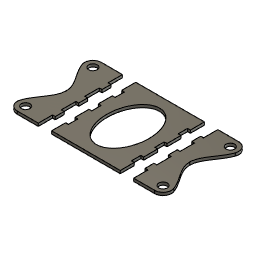
Spuhlenhalter (Autodesk Fusion 360 design; units mm, degrees)
Autodesk Fusion 360 part; units mm, degrees
sketch "Skizze1" plane through (0, 0, 0) normal (0, 1, 0) x (1, 0, 0)
  line L0 (-45, 60) -> (45, 60)
  line L1 (45, 60) -> (45, -60)
  line L2 (45, -60) -> (-45, -60)
  line L3 (-45, -60) -> (-45, 60)
  line L4 (-45, 60) -> (45, -60) construction
  line L5 (45, 60) -> (-45, -60) construction
  line L6 (-45, 60) -> (-49, 60)
  line L7 (-49, 60) -> (-49, 40)
  line L8 (-49, 40) -> (-45, 40)
  line L9 (-45, 40) -> (-45, 60)
  line L10 (-49, 26.6667) -> (-49, 6.6667)
  line L11 (-45, 6.6667) -> (-45, 26.6667)
  line L12 (-45, 26.6667) -> (-49, 26.6667)
  line L13 (-49, 6.6667) -> (-45, 6.6667)
  line L14 (-49, -6.6667) -> (-49, -26.6667)
  line L15 (-45, -26.6667) -> (-45, -6.6667)
  line L16 (-45, -6.6667) -> (-49, -6.6667)
  line L17 (-49, -26.6667) -> (-45, -26.6667)
  line L18 (-49, -40) -> (-49, -60)
  line L19 (-45, -60) -> (-45, -40)
  line L20 (-45, -40) -> (-49, -40)
  line L21 (-49, -60) -> (-45, -60)
  line L22 (0, -1.75) -> (0, -22.5)
  line L23 (45, -40) -> (49, -40)
  line L24 (45, 60) -> (49, 60)
  line L25 (45, 6.6667) -> (45, 26.6667)
  line L26 (49, -26.6667) -> (45, -26.6667)
  line L27 (49, 40) -> (45, 40)
  line L28 (49, -60) -> (45, -60)
  line L29 (45, -60) -> (45, -40)
  line L30 (45, -60) -> (45, 60)
  line L31 (45, 26.6667) -> (49, 26.6667)
  line L32 (49, 6.6667) -> (45, 6.6667)
  line L33 (49, -6.6667) -> (49, -26.6667)
  line L34 (49, 60) -> (49, 40)
  line L35 (45, -6.6667) -> (49, -6.6667)
  line L36 (49, -40) -> (49, -60)
  line L37 (45, -26.6667) -> (45, -6.6667)
  line L38 (45, 40) -> (45, 60)
  line L39 (49, 26.6667) -> (49, 6.6667)
  ellipse E0 centre (0, 0) end of major axis (0, -45) minor radius 30
  line L40 (0, 45) -> (0, -45)
  line L41 (-30, 0) -> (30, 0)
  dimension "d1" = 90
  dimension "d2" = 120
  dimension "d3" = 4
  dimension "d4" = 20
  dimension "d7" = 0
  dimension "d8" = -100
  dimension "d9" = 60
  dimension "d10" = 45
  constraint horizontal L0
  constraint perpendicular L0 L1
  constraint parallel L0 L2
  constraint parallel L1 L3
  constraint coincident L4 E0.centre
  constraint coincident L5 E0.centre
  constraint coincident E0.centre origin
  constraint horizontal L6
  constraint vertical L7
  constraint horizontal L8
  constraint vertical L9
  constraint symmetric L0.start L22 L0.end
  constraint symmetric L2.end L22 L1.end
  constraint symmetric L6.end L22 L24.end
  constraint symmetric L7.end L22 L27.start
  constraint symmetric L8.end L22 L27.end
  constraint symmetric L11.start L22 L25.start
  constraint symmetric L10.start L22 L31.end
  constraint symmetric L10.end L22 L32.start
  constraint symmetric L11.end L22 L25.end
  constraint symmetric L15.start L22 L26.end
  constraint symmetric L14.start L22 L33.start
  constraint symmetric L14.end L22 L26.start
  constraint symmetric L15.end L22 L35.start
  constraint symmetric L18.start L22 L23.end
  constraint symmetric L18.end L22 L28.start
  constraint symmetric L19.end L22 L23.start
  constraint vertical L40
  constraint coincident E0 L40.start
  constraint coincident E0 L40.end
  constraint coincident E0 L41.start
  constraint coincident E0 L41.end
  measures "d1" distance of L1.end L2.end
  measures "d2" distance of L0.end L1.end
  measures "d3" distance of L0.start L6.end
  measures "d4" distance of L0.start L8.end
  measures "d10" distance of E0.centre L40.start
extrude "Extrusion1" add sketch "Skizze1" along normal blind 4 makes body 1
sketch "Skizze2" plane through (0, 0, 0) normal (0, 1, 0) x (1, 0, 0)
  line L0 (-68, 0) -> (-68, 60)
  line L1 (-68, 60) -> (-98, 60)
  arc A0 (-98, 60) -> (-109.2376, 43.791) centre (-98, 48) ccw
  line L2 (-68, 0) -> (-88, 0)
  spline S0 degree 5 poles (-109.2376, 43.791) (-108.5645, 41.9938) (-107.0336, 38.4213) (-104.1836, 33.1279) (-99.539, 26.1758) (-93.573, 17.5532) (-89.8635, 10.6152) (-88.339, 5.3417) (-88, 1.7871) (-88, 0) knots 0 0 0 0 0 0 0.2 0.4 0.6 0.8 1 1 1 1 1 1
  line L3 (-111.0492, 48.6279) -> (-107.4261, 38.9542)
  line L4 (-88, 4.59) -> (-88, -4.59)
  line L5 (49, 60) -> (-49, 60)
  circle A1 centre (-98, 48) radius 6.1
  line L6 (-68, 0) -> (-64, 0)
  line L7 (-64, 0) -> (-64, 6.3667)
  line L8 (-64, 6.3667) -> (-68, 6.3667)
  line L9 (-68, 6.3667) -> (-68, 0)
  line L10 (-68, 26.9667) -> (-64, 26.9667)
  line L11 (-64, 26.9667) -> (-64, 39.7)
  line L12 (-64, 39.7) -> (-68, 39.7)
  line L13 (-68, 39.7) -> (-68, 26.9667)
  line L14 (-49, 6.6667) -> (-45, 6.6667)
  line L15 (-45, 26.6667) -> (-49, 26.6667)
  line L16 (-49, 40) -> (-45, 40)
  line L17 (1.75, 0) -> (22.5, 0)
  line L18 (-64, -26.9667) -> (-64, -39.7)
  line L19 (-68, -6.3667) -> (-68, 0)
  line L20 (-64, -39.7) -> (-68, -39.7)
  line L21 (-68, -60) -> (-98, -60)
  line L22 (-111.0492, -48.6279) -> (-107.4261, -38.9542)
  line L23 (-88, -4.59) -> (-88, 4.59)
  line L24 (-68, 0) -> (-88, 0)
  line L25 (-64, 0) -> (-64, -6.3667)
  spline S1 degree 5 poles (-109.2376, -43.791) (-108.5645, -41.9938) (-107.0336, -38.4213) (-104.1836, -33.1279) (-99.539, -26.1758) (-93.573, -17.5532) (-89.8635, -10.6152) (-88.339, -5.3417) (-88, -1.7871) (-88, 0) knots 0 0 0 0 0 0 0.2 0.4 0.6 0.8 1 1 1 1 1 1
  line L26 (-111.0492, -48.6279) -> (-107.4261, -38.9542)
  line L27 (-88, -4.59) -> (-88, 4.59)
  line L28 (-68, -39.7) -> (-68, -26.9667)
  line L29 (-68, 0) -> (-68, -60)
  circle A2 centre (-98, -48) radius 6.1
  arc A3 (-109.2376, -43.791) -> (-98, -60) centre (-98, -48) ccw
  line L30 (-68, 0) -> (-64, 0)
  line L31 (-64, -6.3667) -> (-68, -6.3667)
  line L32 (-68, -26.9667) -> (-64, -26.9667)
  line L33 (-49, 60) -> (-49, 40)
  dimension "d13" = 12.2
  dimension "d14" = 12
  dimension "d15" = 20
  dimension "d18" = 30
  dimension "d19" = 4
  dimension "d20" = 0.3
  dimension "d21" = 0.3
  dimension "d22" = 0.3
  dimension "d27" = 15
  constraint vertical L0
  constraint perpendicular L0 L1
  constraint tangent L1 A0
  constraint perpendicular L0 L2
  constraint midpoint A0.end L3
  constraint tangent A0 L3
  constraint midpoint L2.end L4
  constraint perpendicular L2 L4
  constraint collinear L1 L5
  constraint concentric A0 A1
  constraint coincident origin L2
  constraint horizontal L6
  constraint vertical L7
  constraint horizontal L8
  constraint vertical L9
  constraint horizontal L10
  constraint vertical L11
  constraint horizontal L12
  constraint vertical L13
  constraint coincident L0 L10.start
  constraint collinear L7 L11
  constraint symmetric L0.start L17 L2.start
  constraint symmetric L0.end L17 L21.start
  constraint symmetric L1.end L17 L21.end
  constraint symmetric A0.end L17 S1.start
  constraint symmetric A0 L17 A3
  constraint symmetric L2.end L17 S0.end
  constraint symmetric L3.start L17 L22.start
  constraint symmetric L3.end L17 L22.end
  constraint symmetric L4.start L17 L4.end
  constraint symmetric L4.end L17 L4.start
  constraint symmetric A1 L17 A2
  constraint symmetric L6.end L17 L7.start
  constraint symmetric L7.end L17 L25.end
  constraint symmetric L8.end L17 L19.start
  constraint symmetric L10.start L17 L28.end
  constraint symmetric L10.end L17 L18.start
  constraint symmetric L11.end L17 L18.end
  constraint symmetric L12.end L17 L20.end
  measures "d13" diameter of A1
  measures "d14" radius of A0
  measures "d15" distance of L0.start L2.end
  measures "d18" distance of L0 A0.centre
  measures "d19" distance of L7.end L8.end
  measures "d20" distance of L8 L14
  measures "d21" distance of L10 L15
  measures "d22" distance of L12 L16
  measures "d27" distance of L11 L33
extrude "Extrusion2" add sketch "Skizze2" along normal blind 4 separate body makes body 2
mirror "Spiegeln1" about plane through (0, 0, 0) normal (1, 0, 0) of bodies 2 makes body 3
equation "d21 = d20"
equation "d22 = d20"
